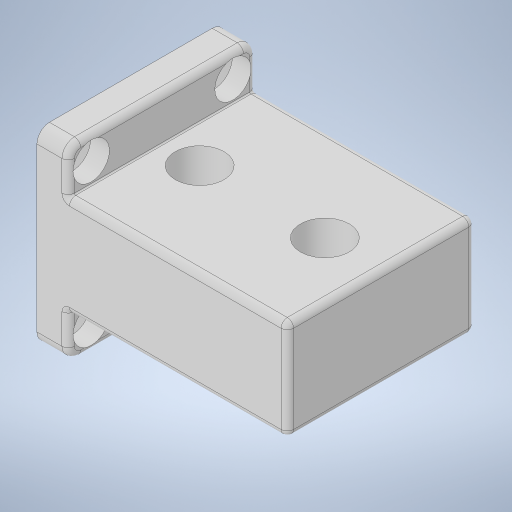
# Autodesk Inventor part: shoulder1_NewPart2
Saved by Autodesk Inventor 2024 (Build 280153000, 153)
## iProperties
Created: 2025-06-25
Part Number: shoulder1_NewPart2
Material: 一般
Document SubType Name: Modeling
Designer: HosodaLab2
Density: 1 g/cm^3
Appearance: 既定
Author: HosodaLab2
Autodesk Inventor part; units mm, degrees
ref_plane "YZ Plane" through (0, 0, 0) normal (1, 0, 0) x (0, 1, 0)
ref_plane "XZ Plane" through (0, 0, 0) normal (0, 1, 0) x (-1, 0, 0)
ref_plane "XY Plane" through (0, 0, 0) normal (0, 0, 1) x (1, 0, 0)
sketch "スケッチ1" plane through (0, 0, 0) normal (0, 1, 0) x (-1, 0, 0)
  line L0 (0, 0) -> (-30, 0)
  line L1 (-30, 0) -> (-30, -30)
  line L2 (-30, -30) -> (0, -30)
  line L3 (0, -30) -> (0, 0)
  dimension "d0" = 30
  dimension "d1" = 30
  constraints: 8 end point, 2 parallel, 1 horizontal, 1 perpendicular
  measures "d0" distance of L2.end L1.end
  measures "d1" distance of L1.end L0.end
extrude "押し出し1" add sketch "スケッチ1" along normal blind 5
sketch "スケッチ2" plane through (0, 5, 0) normal (0, 1, 0) x (1, 0, 0)
  line L0 (30, 0) -> (30, 30) projected
  line L1 (30, 30) -> (0, 30) projected
  line L2 (0, 30) -> (30, 0) construction
  line L3 (30, 30) -> (0, 0) construction
  circle A0 centre (15, 15) radius 16 construction
  point P0 (26.3137, 26.3137)
  point P1 (26.3137, 3.6863)
  point P2 (3.6863, 3.6863)
  point P3 (3.6863, 26.3137)
  point P4 (15, 15)
  dimension "d12" = 32
  dimension "d76" = 0
  constraints: 4 end point, 4 point on circle, 4 point on line, 2 midpoint, 1 centre point, 1 perpendicular
  measures "d12" diameter of A0
  measures "d76" distance of point (15, 15) A0.centre
hole "穴2" at (26.3137, 5, -26.3137) at (26.3137, 5, -3.6863) at (3.6863, 5, -3.6863) at (3.6863, 5, -26.3137) direction (0, -1, 0) diameter 3.2 end through all
sketch "スケッチ3" plane through (0, 5, 0) normal (0, 1, 0) x (1, 0, 0)
  circle A0 centre (26.3137, 3.6863) radius 1.6 projected
  circle A1 centre (3.6863, 3.6863) radius 1.6 projected
  circle A2 centre (3.6863, 26.3137) radius 1.6 projected
  circle A3 centre (26.3137, 26.3137) radius 1.6 projected
  point P0 (0, 0)
  constraints: 4 coincident
hole "穴3" at (26.3137, 5, -3.6863) at (3.6863, 5, -3.6863) at (3.6863, 5, -26.3137) at (26.3137, 5, -26.3137) direction (0, -1, 0) diameter 5.8 depth 3 tip angle 118
sketch "スケッチ4" plane through (0, 5, 0) normal (0, 1, 0) x (1, 0, 0)
  line L0 (0, 30) -> (0, 0) projected
  line L1 (30, 0) -> (30, 30) projected
  line L2 (0, 7) -> (30, 7)
  line L3 (30, 7) -> (30, 23)
  line L4 (30, 23) -> (0, 23)
  line L5 (0, 23) -> (0, 7)
  line L6 (0, 0) -> (30, 0) projected
  point P0 (0, 23)
  dimension "d27" = 16
  dimension "d28" = 7
  constraints: 8 end point, 2 parallel, 2 point on line, 1 horizontal, 1 perpendicular
  measures "d27" distance between parallel lines of L4 L2
  measures "d28" distance between parallel lines of L6 L2
extrude "押し出し2" add sketch "スケッチ4" along normal blind 35 contours L4 L1 L2 L0
fillet "フィレット6" radius 2 4 edges at (30, 2.5, 0) (0, 2.5, 0) (0, 2.5, -30) (30, 2.5, -30)
sketch "スケッチ8" plane through (0, 5, -7) normal (0, 0, 1) x (1, 0, 0)
  line L0 (0, 35) -> (30, 35) projected
  line L1 (2, 0) -> (28, 0) projected
  point P0 (0, -5)
  point P1 (15, 6)
  point P2 (15, 35)
  point P3 (3.089, 0)
  point P4 (23.911, 0)
  dimension "d61" = 6
  constraints: 1 midpoint, 1 vertical alignment
  measures "d61" distance from line of L1 point (15, 6)
hole "穴6" at (15, 11, -7) direction (0, 0, -1) diameter 7.8 end through all
fillet "フィレット7" [suppressed]
fillet "フィレット8" radius 0.2 2 edges at (15, 5, -23) (15, 5, -7)
fillet "フィレット9" radius 1 22 edges at (15, 40, -23) (15, 40, -7) (30, 5.0586, -23.0586) (30, 5, -25.6) (29.4142, 5, -29.4142) (15, 5, -30) (0.5858, 5, -29.4142) (0, 5, -25.6) (0, 5.0586, -23.0586) (0, 22.6, -23) (30, 22.6, -23) (0, 5.0586, -6.9414) (0, 5, -4.4) (0.5858, 5, -0.5858) (15, 5, 0) (29.4142, 5, -0.5858) (30, 5, -4.4) (30, 5.0586, -6.9414) (30, 22.6, -7) (0, 22.6, -7) (0, 40, -15) (30, 40, -15)
fillet "フィレット10" [suppressed]
sketch "スケッチ10" plane through (29, 5.2, -23) normal (0, 0, -1) x (-1, 0, 0)
  line L0 (0, 34.8) -> (28, 34.8) construction
  circle A0 centre (14, 5.8) radius 3.9 construction
  line L1 (14, 34.8) -> (14, 5.8) construction
  arc A1 (9, 31) -> (0, 22) centre (9, 22) ccw construction
  line L2 (14, 5.8) -> (14, 32.2764) construction
  circle A2 centre (14, 5.8) radius 20 construction
  point P0 (29, -5.2)
  point P1 (9, 32)
  point P2 (19, 32)
  point P3 (14, 25.8)
  point P4 (-1, 32)
  point P5 (29, 32)
  dimension "d85" = 40
  dimension "d84" = 0
  constraints: 4 end point, 2 point on circle, 1 centre point, 1 coincident, 1 point on line, 1 vertical, 1 vertical alignment, 4 other
  measures "d84" distance between parallel lines of L1 L2
hole "穴7" at (15, 31, -23) direction (0, 0, 1) diameter 7.8 end through all
